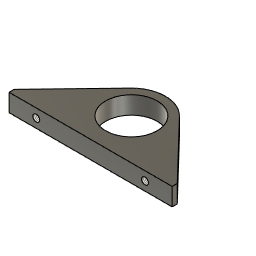
Mancal homemade v3 (Autodesk Fusion 360 design; units mm, degrees)
Autodesk Fusion 360 part; units mm, degrees
sketch "Esboço1" plane through (0, 0, 0) normal (0, 0, 1) x (1, 0, 0)
  circle A0 centre (0, 0) radius 9.5
  circle A1 centre (0, 0) radius 12.5
  line L0 (-30, 22.0941) -> (-30, -26.9412) construction
  line L1 (-41.3447, -13.125) -> (30, -13.125) construction
  line L2 (-30, -13.125) -> (-9.0024, 8.6722)
  line L3 (-30, -13.125) -> (-30, -15)
  line L4 (-30, -15) -> (0, -15)
  line L5 (0, 0) -> (0, -30) construction
  line L6 (30, -13.125) -> (9.0024, 8.6722)
  line L7 (30, -13.125) -> (30, -15)
  line L8 (30, -15) -> (0, -15)
  dimension "d1" = 25
  dimension "d2" = 19
  dimension "d3" = 30
  dimension "d4" = 13.125
  dimension "d6" = 1.875
  constraint coincident A0.centre A1.centre
  constraint concentric A0 A1
  constraint vertical L0
  constraint perpendicular L0 L1
  constraint coincident L0 L2.start
  constraint tangent A1 L2
  constraint coincident L1 L2.start
  constraint coincident A1 L2.end
  constraint coincident L0 L3.end
  constraint perpendicular L3 L4
  constraint perpendicular L1 L5
  constraint symmetric L2.start L5 L1.end
  constraint symmetric L2.end L5 L6.end
  constraint symmetric L3.end L5 L7.end
  constraint symmetric L4.end L5 L8.end
  measures "d1" diameter of A1
  measures "d2" diameter of A0
  measures "d3" distance of A0.centre L0
  measures "d4" distance of A0.centre L1
  measures "d6" distance of L2.start L3.end
extrude "Extrusão1" add sketch "Esboço1" along normal blind 6.5
sketch "Esboço2" plane through (0, -15, 0) normal (0, -1, 0) x (1, 0, 0)
  line L0 (-30, 0) -> (30, 0)
  line L1 (30, 0) -> (30, 6.5)
  line L2 (30, 6.5) -> (-30, 6.5)
  line L3 (-30, 6.5) -> (-30, 0)
  line L4 (0, 0) -> (0, 15) construction
  line L5 (-20, 3.25) -> (20, 3.25) construction
  circle A0 centre (-20, 3.25) radius 1.5
  circle A1 centre (20, 3.25) radius 1.5
  dimension "d9" = 20
  dimension "d10" = 20
  dimension "d11" = 3.25
  dimension "d12" = 3
  constraint coincident L4.start origin
  constraint perpendicular L2 L4
  constraint perpendicular L4 L5
  constraint coincident L5.start A0.centre
  constraint symmetric L4 A0 A1
  measures "d9" horizontal distance of L4.start L5.start
  measures "d10" horizontal distance of L4.start L5.end
  measures "d11" distance of L0 L5
  measures "d12" diameter of A0
extrude "Extrusão2" cut sketch "Esboço2" against normal blind 8 contours A0 | A1
thread "Rosca1" "ISO Metric profile 3.0 M3x0.5 6H" major diameter 3.086 minor diameter 2.529 pitch 0.5 angle 60 resizes the face on face at (21.4925, -9.6667, 3.1006) on face at (-18.5075, -9.6667, 3.1006)
